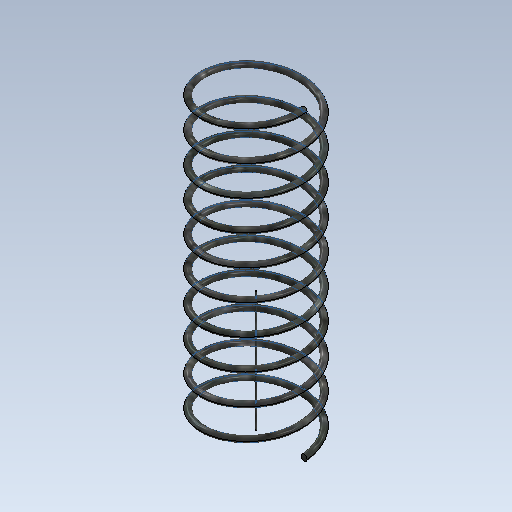
# Autodesk Inventor part: タミヤダンパー9
Saved by Autodesk Inventor 2020 (Build 240168000, 168)
## iProperties
Created: 2020-04-10
Part Number: タミヤダンパー9
Material: 鋼
Document SubType Name: Modeling
Designer: happy
Mass: 40.8 g
Surface Area: 15.9724 cm^2
Volume: 0.395412 cm^3
Density: 103.183 g/cm^3
Appearance: プレート
Author: happy
Autodesk Inventor part; units mm, degrees
ref_plane "YZ Plane" through (0, 0, 0) normal (1, 0, 0) x (0, 1, 0)
ref_plane "XZ Plane" through (0, 0, 0) normal (0, 1, 0) x (-1, 0, 0)
ref_plane "XY Plane" through (0, 0, 0) normal (0, 0, 1) x (1, 0, 0)
sketch "スケッチ1" plane through (0, 0, 0) normal (0, 0, 1) x (1, 0, 0)
  line L0 (0, 0) -> (0, 20) construction
  line L1 (0, 20) -> (8, 20) construction
  circle A0 centre (8, 20) radius 0.5
  line L2 (0, 20) -> (0.1, 20)
  line L3 (0.1, 20) -> (0.1, 40)
  line L4 (0.1, 40) -> (0, 40)
  line L5 (0, 40) -> (0, 20)
  dimension "d0" = 1
  dimension "d1" = 8
  dimension "d2" = 20
  dimension "d11" = 0.1
  dimension "d12" = 20
  constraints: 12 end point, 2 parallel, 2 perpendicular, 1 centre point, 1 coincident, 1 horizontal, 1 vertical
  measures "d0" diameter of A0
  measures "d1" distance of L0.end L1.end
  measures "d2" distance of L0.start L0.end
  measures "d11" distance of L4.end L3.end
  measures "d12" distance of L3.end L2.end
coil "コイル1" sketch "スケッチ1" operation add axis through (0, 0, 0) along (0, 1, 0) pitch 5 turns 10 hand right contours A0
revolve "回転1" add sketch "スケッチ1" angle 360 about axis through (0, 40, 0) along (0, -1, 0) contours L5 L4 L3 L2
equation "\"d2\" = d12"
